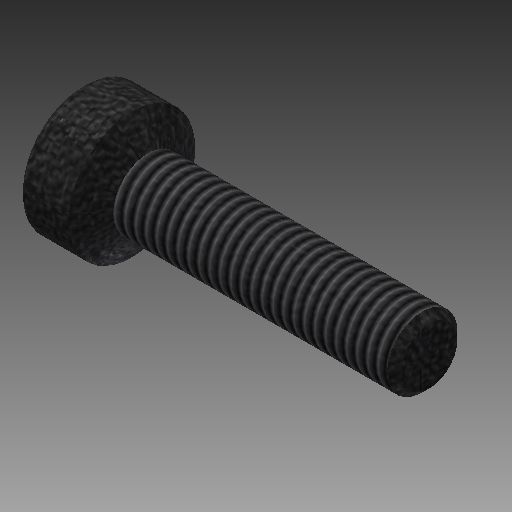
# Autodesk Inventor part: Torx T50 M10 x 1,25
Saved by Autodesk Inventor 2019 (Build 230136000, 136)
## iProperties
Created: 2016-12-14
Part Number: Torx T50 M10 x 1,25
Material: 钢，高强度，低合金
Document SubType Name: Modeling
Designer: Catweazle
Density: 7.85 g/cm^3
Appearance: Schwarz - Guss
Author: Catweazle
Autodesk Inventor part; units mm, degrees
ref_plane "YZ Plane" through (0, 0, 0) normal (1, 0, 0) x (0, 1, 0)
ref_plane "XZ Plane" through (0, 0, 0) normal (0, 1, 0) x (-1, 0, 0)
ref_plane "XY Plane" through (0, 0, 0) normal (0, 0, 1) x (1, 0, 0)
sketch "Skizze1" plane through (0, 0, 0) normal (0, 0, 1) x (1, 0, 0)
  line L0 (-9.8619, 0) -> (59.1713, 0) projected
  line L1 (0, -1.8) -> (0, 10.8) projected
  line L2 (0, 0) -> (0, 9)
  line L3 (0, 9) -> (7, 9)
  line L4 (7, 9) -> (9.3094, 5)
  line L5 (9.3094, 5) -> (49.3094, 5)
  line L6 (49.3094, 5) -> (49.3094, 0)
  line L7 (49.3094, 0) -> (0, 0)
  dimension "d0" = 18
  dimension "d1" = 7
  dimension "d3" = 10
  dimension "d4" = 40
  dimension "d16" = 60
  constraints: 12 end point, 2 point on line, 1 collinear, 1 horizontal, 1 parallel, 1 perpendicular
  measures "d0" diameter of L3 L0
  measures "d1" distance of L2.end L3.end
  measures "d3" diameter of L5 L0
  measures "d4" distance from line of L4.end L6
  measures "d16" angle of L5 L4
revolve "Umdrehung1" add sketch "Skizze1" angle 360 about axis through (-10, 0, 0) along (1, 0, 0)
chamfer "Fase1" distance 1 angle 45 1 edges at (49.3094, -5, 0)
chamfer "Fase2" distance 0.5 angle 45 1 edges at (0, -9, 0)
thread "Gewinde1" size "M10x1.5" class "6g" standard "ANSI Metric M Profile" full length
sketch "Skizze2" plane through (0, 0, 0) normal (-1, 0, 0) x (0, 0, 1)
  spline S0 degree 3 poles (0.7512, 3.8741) (0.7506, 3.8768) (0.75, 3.8795) (0.7227, 3.995) (0.6691, 4.1023) (0.5302, 4.2738) (0.4382, 4.3487) (0.229, 4.4493) (0.1117, 4.475) (0, 4.475) knots 2.407009 2.407009 2.407009 2.407009 2.415407 2.415407 2.762565 2.762565 3.097556 3.097556 3.432546 3.432546 3.432546 3.432546
  spline S1 degree 3 poles (0, 4.475) (-0.1117, 4.475) (-0.229, 4.4493) (-0.4383, 4.3487) (-0.5302, 4.2739) (-0.6692, 4.1024) (-0.7228, 3.995) (-0.7501, 3.8795) (-0.7507, 3.8768) (-0.7514, 3.8741) knots 3.432546 3.432546 3.432546 3.432546 3.767537 3.767537 4.102528 4.102528 4.449685 4.449685 4.458083 4.458083 4.458083 4.458083
  spline S2 degree 3 poles (-0.7514, 3.8741) (-0.7825, 3.7367) (-0.83, 3.604) (-0.9596, 3.341) (-1.058, 3.1943) (-1.298, 2.9367) (-1.4398, 2.8257) (-1.7272, 2.6597) (-1.8942, 2.5924) (-2.2374, 2.5134) (-2.4136, 2.5016) (-2.7062, 2.5208) (-2.8448, 2.546) (-2.9794, 2.5877) knots 7.439135 7.439135 7.439135 7.439135 7.853901 7.853901 8.351764 8.351764 8.849626 8.849626 9.347489 9.347489 9.845351 9.845351 10.260117 10.260117 10.260117 10.260117
  spline S3 degree 3 poles (-2.9794, 2.5877) (-2.982, 2.5886) (-2.9847, 2.5894) (-3.0984, 2.6235) (-3.2181, 2.6307) (-3.4362, 2.5961) (-3.547, 2.5539) (-3.7387, 2.423) (-3.8196, 2.3342) (-3.8755, 2.2375) knots 2.407009 2.407009 2.407009 2.407009 2.415407 2.415407 2.762565 2.762565 3.097556 3.097556 3.432546 3.432546 3.432546 3.432546
  spline S4 degree 3 poles (-3.8755, 2.2375) (-3.9313, 2.1408) (-3.9677, 2.0263) (-3.9853, 1.7948) (-3.9664, 1.6777) (-3.8873, 1.4716) (-3.8212, 1.3716) (-3.7348, 1.2902) (-3.7328, 1.2882) (-3.7307, 1.2863) knots 3.432546 3.432546 3.432546 3.432546 3.767537 3.767537 4.102528 4.102528 4.449685 4.449685 4.458083 4.458083 4.458083 4.458083
  spline S5 degree 3 poles (-3.7307, 1.2863) (-3.6273, 1.1907) (-3.5361, 1.0832) (-3.3732, 0.8394) (-3.2953, 0.6809) (-3.1922, 0.3442) (-3.167, 0.1659) (-3.1669, -0.166) (-3.1921, -0.3443) (-3.2953, -0.681) (-3.3731, -0.8395) (-3.536, -1.0833) (-3.6272, -1.1908) (-3.7306, -1.2865) knots 7.439135 7.439135 7.439135 7.439135 7.853901 7.853901 8.351764 8.351764 8.849626 8.849626 9.347489 9.347489 9.845351 9.845351 10.260117 10.260117 10.260117 10.260117
  spline S6 degree 3 poles (-3.7306, -1.2865) (-3.7327, -1.2884) (-3.7347, -1.2903) (-3.8211, -1.3717) (-3.8872, -1.4717) (-3.9663, -1.6778) (-3.9852, -1.7948) (-3.9677, -2.0263) (-3.9313, -2.1408) (-3.8755, -2.2375) knots 2.407009 2.407009 2.407009 2.407009 2.415407 2.415407 2.762565 2.762565 3.097556 3.097556 3.432546 3.432546 3.432546 3.432546
  spline S7 degree 3 poles (-3.8755, -2.2375) (-3.8196, -2.3342) (-3.7387, -2.4229) (-3.547, -2.5539) (-3.4362, -2.5961) (-3.2182, -2.6306) (-3.0984, -2.6233) (-2.9848, -2.5893) (-2.9821, -2.5884) (-2.9794, -2.5876) knots 3.432546 3.432546 3.432546 3.432546 3.767537 3.767537 4.102528 4.102528 4.449685 4.449685 4.458083 4.458083 4.458083 4.458083
  spline S8 degree 3 poles (-2.9794, -2.5876) (-2.8449, -2.5459) (-2.7062, -2.5206) (-2.4136, -2.5014) (-2.2374, -2.5132) (-1.8942, -2.5923) (-1.7272, -2.6596) (-1.4397, -2.8256) (-1.2979, -2.9365) (-1.0578, -3.1942) (-0.9595, -3.3409) (-0.8298, -3.6039) (-0.7824, -3.7367) (-0.7512, -3.8741) knots 7.439135 7.439135 7.439135 7.439135 7.853901 7.853901 8.351764 8.351764 8.849626 8.849626 9.347489 9.347489 9.845351 9.845351 10.260117 10.260117 10.260117 10.260117
  spline S9 degree 3 poles (-0.7512, -3.8741) (-0.7506, -3.8768) (-0.75, -3.8795) (-0.7227, -3.995) (-0.6691, -4.1023) (-0.5302, -4.2738) (-0.4382, -4.3487) (-0.229, -4.4493) (-0.1117, -4.475) (0, -4.475) knots 2.407009 2.407009 2.407009 2.407009 2.415407 2.415407 2.762565 2.762565 3.097556 3.097556 3.432546 3.432546 3.432546 3.432546
  spline S10 degree 3 poles (0, -4.475) (0.1117, -4.475) (0.229, -4.4493) (0.4382, -4.3487) (0.5302, -4.2738) (0.6691, -4.1023) (0.7227, -3.995) (0.75, -3.8795) (0.7506, -3.8768) (0.7512, -3.8741) knots 3.432546 3.432546 3.432546 3.432546 3.767537 3.767537 4.102528 4.102528 4.449685 4.449685 4.458083 4.458083 4.458083 4.458083
  spline S11 degree 3 poles (0.7512, -3.8741) (0.7824, -3.7367) (0.8298, -3.604) (0.9595, -3.341) (1.0579, -3.1943) (1.2979, -2.9366) (1.4397, -2.8257) (1.7272, -2.6597) (1.8942, -2.5924) (2.2374, -2.5134) (2.4136, -2.5015) (2.7062, -2.5208) (2.8448, -2.546) (2.9794, -2.5877) knots 7.439135 7.439135 7.439135 7.439135 7.853901 7.853901 8.351764 8.351764 8.849626 8.849626 9.347489 9.347489 9.845351 9.845351 10.260117 10.260117 10.260117 10.260117
  spline S12 degree 3 poles (2.9794, -2.5877) (2.982, -2.5886) (2.9847, -2.5894) (3.0984, -2.6235) (3.2181, -2.6307) (3.4362, -2.5961) (3.547, -2.5539) (3.7387, -2.423) (3.8196, -2.3342) (3.8755, -2.2375) knots 2.407009 2.407009 2.407009 2.407009 2.415407 2.415407 2.762565 2.762565 3.097556 3.097556 3.432546 3.432546 3.432546 3.432546
  spline S13 degree 3 poles (3.8755, -2.2375) (3.9313, -2.1408) (3.9677, -2.0263) (3.9852, -1.7948) (3.9663, -1.6778) (3.8872, -1.4717) (3.8211, -1.3717) (3.7347, -1.2903) (3.7327, -1.2884) (3.7306, -1.2865) knots 3.432546 3.432546 3.432546 3.432546 3.767537 3.767537 4.102528 4.102528 4.449685 4.449685 4.458083 4.458083 4.458083 4.458083
  spline S14 degree 3 poles (3.7306, -1.2865) (3.6272, -1.1908) (3.536, -1.0833) (3.3731, -0.8395) (3.2953, -0.681) (3.1921, -0.3443) (3.1669, -0.166) (3.167, 0.1659) (3.1922, 0.3442) (3.2953, 0.6809) (3.3732, 0.8394) (3.5361, 1.0832) (3.6273, 1.1907) (3.7307, 1.2863) knots 7.439135 7.439135 7.439135 7.439135 7.853901 7.853901 8.351764 8.351764 8.849626 8.849626 9.347489 9.347489 9.845351 9.845351 10.260117 10.260117 10.260117 10.260117
  spline S15 degree 3 poles (3.7307, 1.2863) (3.7328, 1.2882) (3.7348, 1.2902) (3.8212, 1.3716) (3.8873, 1.4716) (3.9664, 1.6777) (3.9853, 1.7948) (3.9677, 2.0263) (3.9313, 2.1408) (3.8755, 2.2375) knots 2.407009 2.407009 2.407009 2.407009 2.415407 2.415407 2.762565 2.762565 3.097556 3.097556 3.432546 3.432546 3.432546 3.432546
  spline S16 degree 3 poles (3.8755, 2.2375) (3.8196, 2.3342) (3.7387, 2.423) (3.547, 2.5539) (3.4362, 2.5961) (3.2181, 2.6307) (3.0984, 2.6235) (2.9847, 2.5894) (2.982, 2.5886) (2.9794, 2.5877) knots 3.432546 3.432546 3.432546 3.432546 3.767537 3.767537 4.102528 4.102528 4.449685 4.449685 4.458083 4.458083 4.458083 4.458083
  spline S17 degree 3 poles (2.9794, 2.5877) (2.8448, 2.546) (2.7062, 2.5208) (2.4136, 2.5015) (2.2374, 2.5134) (1.8942, 2.5924) (1.7272, 2.6597) (1.4397, 2.8257) (1.2979, 2.9366) (1.0579, 3.1943) (0.9595, 3.341) (0.8298, 3.604) (0.7824, 3.7367) (0.7512, 3.8741) knots 7.439135 7.439135 7.439135 7.439135 7.853901 7.853901 8.351764 8.351764 8.849626 8.849626 9.347489 9.347489 9.845351 9.845351 10.260117 10.260117 10.260117 10.260117
  point P0 (0, 0)
  point P1 (0, 0)
  point P2 (0, 0)
  constraints: 36 other
extrude "Extrusion1" cut sketch "Skizze2" against normal blind 6
